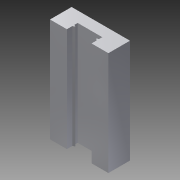
# Autodesk Inventor part: slide
Saved by Autodesk Inventor 2015 (Build 190159000, 159)
## iProperties
Created: 2015-01-29
Part Number: slide
Material: Generic
Document SubType Name: Modeling
Designer: Joseph
Density: 1 g/cm^3
Appearance: Aluminum - Flat
Author: Joseph
Autodesk Inventor part; units mm, degrees
ref_plane "YZ Plane" through (0, 0, 0) normal (1, 0, 0) x (0, 1, 0)
ref_plane "XZ Plane" through (0, 0, 0) normal (0, 1, 0) x (-1, 0, 0)
ref_plane "XY Plane" through (0, 0, 0) normal (0, 0, 1) x (1, 0, 0)
sketch "Sketch1" plane through (0, 0, 0) normal (0, 0, 1) x (1, 0, 0)
  line L0 (13.5, 5) -> (-13.5, 5)
  line L1 (-13.5, 5) -> (-13.5, -5)
  line L2 (13.5, -5) -> (13.5, 5)
  line L3 (13.5, 5) -> (-13.5, -5) construction
  line L4 (-13.5, 5) -> (13.5, -5) construction
  line L5 (-5.6959, -5) -> (-5.6959, -2.5129)
  line L6 (-5.6959, -2.5129) -> (-4.75, -2)
  line L7 (-4.75, -2) -> (-5.6959, -1.4871)
  line L8 (-5.6959, -1.4871) -> (-5.6959, 0)
  line L9 (-5.6959, 0) -> (5.6959, 0)
  line L10 (5.6959, 0) -> (5.6959, -1.4871)
  line L11 (5.6959, -1.4871) -> (4.75, -2)
  line L12 (4.75, -2) -> (5.6959, -2.5129)
  line L13 (5.6959, -2.5129) -> (5.6959, -5)
  line L14 (-13.5, -5) -> (-5.6959, -5)
  line L15 (5.6959, -5) -> (13.5, -5)
  point P0 (0, 0)
  dimension "d0" = 27
  dimension "d1" = 10
  dimension "d2" = 5
  dimension "d3" = 9.5
  dimension "d4" = 7
  dimension "d5" = 5
  constraints: 32 end point, 6 equal length, 4 parallel, 4 point on line, 3 perpendicular, 2 midpoint, 1 horizontal, 1 vertical
  measures "d0" distance of L2.start L1.end
  measures "d1" distance of L1.end L0.end
  measures "d2" distance between parallel lines of L0 L9
  measures "d3" distance of L11.end L6.end
  measures "d4" distance from line of L0 L6.end
  measures "d5" distance between parallel lines of L14 L9
extrude "Extrusion1" add sketch "Sketch1" along normal blind 48
sketch "Sketch2" plane through (-13.5, 5, 0) normal (0, 1, 0) x (1, 0, 0)
  line L0 (23.9186, -34) -> (3.9186, -34) construction
  line L1 (3.9186, -34) -> (3.9186, -14) construction
  line L2 (3.9186, -14) -> (23.9186, -14) construction
  line L3 (23.9186, -14) -> (23.9186, -34) construction
  line L4 (23.9186, -34) -> (3.9186, -14) construction
  line L5 (3.9186, -34) -> (23.9186, -14) construction
  point P0 (13.5, 0)
  point P1 (13.9186, -24)
  dimension "d8" = 20
  dimension "d9" = 20
  constraints: 12 end point, 4 coincident, 2 midpoint, 2 parallel, 1 horizontal, 1 perpendicular
  measures "d8" distance of L1.end L2.end
  measures "d9" distance of L0.end L1.end
hole "Hole1" at (-9.5814, 5, 34) at (-9.5814, 5, 14) at (10.4186, 5, 14) at (10.4186, 5, 34) direction (0, -1, 0) diameter 2.459 depth 3.5 tip angle 118 thread size "M3x0.5" class "6H" standard "ANSI Metric M Profile"
body "Solid1"
